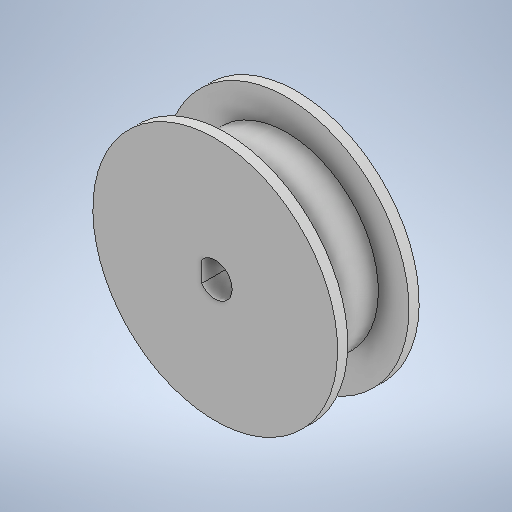
# Autodesk Inventor part: Pulley
Saved by Autodesk Inventor 2025 (Build 290162000, 162)
## iProperties
Created: 2024-10-28
Part Number: Pulley
Material: Generic
Document SubType Name: Modeling
Designer: liaco
Density: 1 g/cm^3
Appearance: Default
Mass: 6.43084 g
Surface Area: 35.5471 cm^2
Volume: 6.43084 cm^3
Author: liaco
Autodesk Inventor part; units mm, degrees
ref_plane "YZ Plane" through (0, 0, 0) normal (1, 0, 0) x (0, 1, 0)
ref_plane "XZ Plane" through (0, 0, 0) normal (0, 1, 0) x (-1, 0, 0)
ref_plane "XY Plane" through (0, 0, 0) normal (0, 0, 1) x (1, 0, 0)
sketch "Sketch2" plane through (0, 0, 0) normal (1, 0, 0) x (0, 1, 0)
  line L0 (0, 6) -> (18, 6)
  line L1 (18, 6) -> (18, 4.5)
  line L2 (18, 4.5) -> (13.5, 4.5)
  line L3 (13.5, 4.5) -> (13.5, -4.5)
  line L4 (13.5, -4.5) -> (18, -4.5)
  line L5 (18, -4.5) -> (18, -6)
  line L6 (18, -6) -> (0, -6)
  line L7 (0, -6) -> (0, 6)
  point P0 (0, 0)
  point P1 (18, -5.25)
  dimension "d0" = 18
  dimension "d1" = 4.5
  dimension "d2" = 18
  dimension "d3" = 12
  dimension "d4" = 6
  dimension "d5" = 1.5
  constraints: 16 end point, 6 perpendicular, 2 point on line, 1 collinear, 1 horizontal, 1 midpoint
  measures "d0" distance of L5.end L6.end
  measures "d1" distance of L1.end L2.end
  measures "d2" horizontal distance of point (18, -5.25) point (0, 0)
  measures "d3" distance of L6.end L0.start
  measures "d4" distance of L6.end point (0, 0)
  measures "d5" distance of L4.end L5.end
revolve "Revolution1" add sketch "Sketch2" angle 360 about axis through (0, 0, -6) along (0, 0, 1)
sketch "Sketch3" plane through (0, 0, 6) normal (0, 0, 1) x (1, 0, 0)
  arc A0 (-2, -1.5) -> (-2, 1.5) centre (0, 0) ccw
  line L0 (-2, 1.5) -> (-2, -1.5)
  point P0 (0, 0)
  dimension "d14" = 5
  dimension "d15" = 3
  constraints: 2 coincident, 2 end point, 2 point on circle, 1 centre point, 1 vertical
  measures "d14" diameter of A0
  measures "d15" distance of L0.start L0.end
extrude "Extrusion1" cut sketch "Sketch3" against normal through all
body "Solid1"
